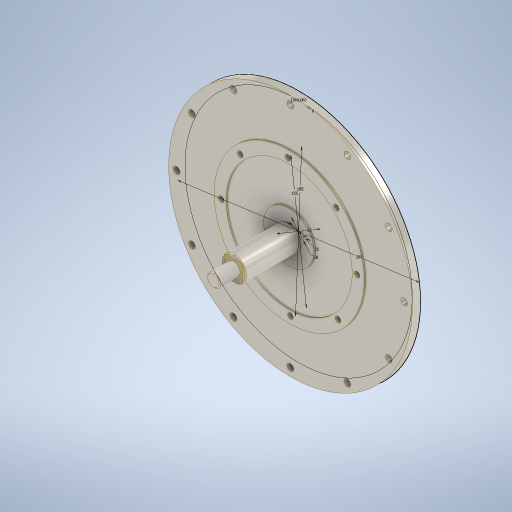
# Autodesk Inventor part: podstawa
Saved by Autodesk Inventor 2023 (Build 270158000, 158)
## iProperties
Created: 2023-03-26
Part Number: podstawa
Material: Tytan
Document SubType Name: Modeling
Designer: krzys
Density: 4.51 g/cm^3
Appearance: Tytan
Mass: 3481.29 g
Surface Area: 1621.76 cm^2
Volume: 771.904 cm^3
Author: krzys
## iProperties of the stored document podstawa_Drukowanie 3D.ipt
Created: 2023-04-25
Part Number: podstawa_Drukowanie 3D
Material: Ogólny
Document SubType Name: Modeling
Designer: krzys
Density: 1 g/cm^3
Appearance: Domyślna
Author: krzys
Autodesk Inventor part; units mm, degrees
ref_plane "YZ Plane" through (0, 0, 0) normal (1, 0, 0) x (0, 1, 0)
ref_plane "XZ Plane" through (0, 0, 0) normal (0, 1, 0) x (-1, 0, 0)
ref_plane "XY Plane" through (0, 0, 0) normal (0, 0, 1) x (1, 0, 0)
sketch "Szkic1" plane through (0, 0, 0) normal (0, 0, 1) x (1, 0, 0)
  circle A0 centre (0, 0) radius 150
  circle A1 centre (0, 0) radius 15
  circle A2 centre (0, 140) radius 4
  circle A3 centre (-70, 121.2436) radius 4
  circle A4 centre (-121.2436, 70) radius 4
  circle A5 centre (-140, 0) radius 4
  circle A6 centre (-121.2436, -70) radius 4
  circle A7 centre (-70, -121.2436) radius 4
  circle A8 centre (0, 0) radius 31
  circle A9 centre (0, -140) radius 4
  circle A10 centre (70, -121.2436) radius 4
  circle A11 centre (0, 0) radius 14
  circle A12 centre (0, 0) radius 12.5
  circle A13 centre (121.2436, -70) radius 4
  circle A14 centre (140, 0) radius 4
  circle A15 centre (121.2436, 70) radius 4
  circle A16 centre (70, 121.2436) radius 4
  circle A17 centre (0, 0) radius 92.5
  circle A18 centre (0, 0) radius 77.5
  dimension "d0" = 300
  dimension "d1" = 30
  dimension "d2" = 8
  dimension "d5" = 360
  dimension "d7" = 62
  dimension "d15" = 28
  dimension "d16" = 25
  dimension "d55" = 185
  dimension "d56" = 155
  constraints: 19 centre point, 7 coincident, 25 other
  measures "d0" diameter of A0
  measures "d1" diameter of A1
  measures "d2" diameter of A2
  measures "d7" diameter of A8
  measures "d15" diameter of A11
  measures "d16" diameter of A12
  measures "d55" diameter of A17
  measures "d56" diameter of A18
extrude "Wyciągnięcie proste1" add sketch "Szkic1" along normal blind 80 contours A1 | A11 | A12
extrude "Wyciągnięcie proste2" add sketch "Szkic1" along normal blind 12 contours A8
ref_plane "Płaszczyzna konstrukcyjna1" through (0, 0, 80) normal (0, 0, 1) x (1, 0, 0)
sketch "Szkic2" plane through (0, 0, 80) normal (0, 0, 1) x (1, 0, 0)
  circle A0 centre (0, 0) radius 8
  dimension "d21" = 16
  constraints: 1 centre point, 1 coincident
  measures "d21" diameter of A0
extrude "Wyciągnięcie proste6" add sketch "Szkic2" along normal blind 25
extrude "Wyciągnięcie proste8" add sketch "Szkic1" along normal blind 10 contours A0 | A18
chamfer "Faza2" distance 1 angle 45 1 edges at (-15, 0, 80)
thread "Gwint2" size "M16x2" class "6g" standard "ANSI Metric M Profile" full length
chamfer "Faza4" distance 1 angle 45 1 edges at (-8, 0, 105)
extrude "Wyciągnięcie proste9" add sketch "Szkic1" along normal blind 11.5 contours A17
sketch "Szkic10" plane through (0, 0, 0) normal (0, 0, -1) x (-1, 0, 0)
  point P0 (-1.558, -83.5832)
hole "Otwór8" at (1.558, -83.5832, 0) direction (0, 0, 1) diameter 6.6 end through all
sketch "Szkic11" plane through (0, 0, 0) normal (0, 0, -1) x (-1, 0, 0)
  point P0 (-60.2039, -58.0006)
hole "Otwór9" at (60.2039, -58.0006, 0) direction (0, 0, 1) diameter 6.6 end through all
sketch "Szkic12" plane through (0, 0, 0) normal (0, 0, -1) x (-1, 0, 0)
  point P0 (-83.5832, 1.558)
hole "Otwór10" at (83.5832, 1.558, 0) direction (0, 0, 1) diameter 6.6 end through all
sketch "Szkic13" plane through (0, 0, 0) normal (0, 0, -1) x (-1, 0, 0)
  point P0 (-58.0006, 60.2039)
hole "Otwór11" at (58.0006, 60.2039, 0) direction (0, 0, 1) diameter 6.6 end through all
sketch "Szkic14" plane through (0, 0, 0) normal (0, 0, -1) x (-1, 0, 0)
  point P0 (1.558, 83.5832)
hole "Otwór12" at (-1.558, 83.5832, 0) direction (0, 0, 1) diameter 6.6 end through all
sketch "Szkic15" plane through (0, 0, 0) normal (0, 0, -1) x (-1, 0, 0)
  point P0 (60.2039, 58.0006)
hole "Otwór13" at (-60.2039, 58.0006, 0) direction (0, 0, 1) diameter 6.6 end through all
sketch "Szkic16" plane through (0, 0, 0) normal (0, 0, -1) x (-1, 0, 0)
  point P0 (83.5832, -1.558)
hole "Otwór14" at (-83.5832, -1.558, 0) direction (0, 0, 1) diameter 6.6 end through all
sketch "Szkic17" plane through (0, 0, 0) normal (0, 0, -1) x (-1, 0, 0)
  point P0 (58.0006, -60.2039)
hole "Otwór15" at (-58.0006, -60.2039, 0) direction (0, 0, 1) diameter 6.6 end through all
